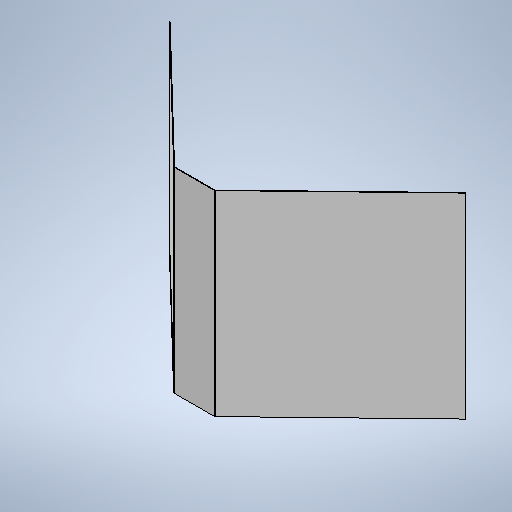
# Autodesk Inventor part: MSC 501 SHEET BELLY MAIN
Saved by Autodesk Inventor 2025 (Build 290162010, 162A)
## iProperties
Created: 2024-04-28
Part Number: MSC 501 SHEET BELLY MAIN
Material: Stainless Steel
Document SubType Name: Sheet Metal
Designer: admin
Density: 8 g/cm^3
Flat Pattern Width: 198.004 cm
Flat Pattern Length: 98 cm
Flat Pattern Area: 19404.3 cm^2
Sheet Metal Rule: Default_mm
Sheet Metal Width: 1980.035 mm
Sheet Metal Length: 980.000 mm
Sheet Metal Area: 1940434.343 mm^2
Appearance: Default
Mass: 46591 g
Surface Area: 39003.5 cm^2
Volume: 5823.88 cm^3
Stock Number: МОО 501 лист брюхо основной
Author: admin
Autodesk Inventor part; units mm, degrees
note: some values were not read from the file. Chosen so that the rebuilt part matches the saved one: flange form of "Plate1".
ref_plane "YZ Plane" through (0, 0, 0) normal (1, 0, 0) x (0, 1, 0)
ref_plane "XZ Plane" through (0, 0, 0) normal (0, 1, 0) x (-1, 0, 0)
ref_plane "XY Plane" through (0, 0, 0) normal (0, 0, 1) x (1, 0, 0)
sketch "Sketch1" plane through (0, 0, 0) normal (0, 0, 1) x (1, 0, 0)
  line L0 (104.168, 1.684) -> (742.0066, 617.6375)
  arc A0 (100, 0) -> (104.168, 1.684) centre (100, 6) ccw
  line L1 (0, 0) -> (100, 0)
  dimension "d25" = 6
  dimension "d48" = 742.0065
  dimension "d49" = 136
  dimension "d50" = 100
  dimension "d51" = 886.7
  measures "d25" radius of A0
  measures "d48" horizontal distance of L1.start L0.end
  measures "d49" angle of L1 L0
  measures "d50" distance of L1.start L1.end
  measures "d51" distance of L0.start L0.end
contour flange "Contour Flange1" sketch "Sketch1" thickness 3 bend radius 3 width 980 along (0, 0, 1) mid plane no both sides no wall seen from (50, 0, 0) lies toward (0, 1, 0) curves L1 A0 L0
bend "Bend1"
corner "Corner1"
mirror "Mirror1" about plane through (0, 0, 0) normal (1, 0, 0)
sketch "Sketch2" plane through (-102.084, 3.842, 980) normal (0.6946584, 0.7193398, 0) x (0.7193398, -0.6946584, 0)
  line L0 (-842.2117, 70.9383) -> (-842.2117, 209.5784) construction
  line L1 (-842.2117, 209.5784) -> (-819.3515, 209.5784) construction
  line L2 (-819.3515, 209.5784) -> (-819.3515, 70.9383) construction
  line L3 (-819.3515, 70.9383) -> (-842.2117, 70.9383) construction
  point P0 (76.1019, 980)
  constraints: 2 other
mark "Mark1"
equation "\"d25\" = Thickness + BendRadius"
equation "\"d7\" = Thickness"
equation "\"d8\" = BendReliefWidth"
equation "\"d9\" = BendReliefDepth"
equation "\"d10\" = MinimumRemnant"
equation "\"d11\" = TransitionRadius"
equation "\"d13\" = BendRadius"
equation "\"d15\" = CornerReliefSize"
equation "\"d16\" = GapSize"
equation "\"d17\" = JacobiRadiusSize"
equation "\"BendRadius\" = Thickness"
equation "\"BendReliefWidth\" = Thickness"
equation "\"BendReliefDepth\" = 0.5 * Thickness"
equation "\"CornerReliefSize\" = 4 * Thickness"
equation "\"MinimumRemnant\" = 2 * Thickness"
equation "\"TransitionRadius\" = BendRadius"
equation "\"JacobiRadiusSize\" = BendRadius"
equation "\"GapSize\" = Thickness"
equation "\"d38\" = d40 + d44"
equation "\"d39\" = d40"
equation "\"d44\" = d40"
equation "\"Thickness\" = 3"
equation "\"d40\" = 3"
body "Solid1"
